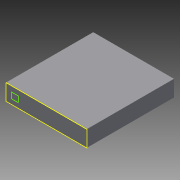
# Autodesk Inventor part: Five Pin Plug
Saved by Autodesk Inventor 2014 (Build 180170000, 170)
## iProperties
Created: 2014-02-26
Part Number: Five Pin Plug
Material: Generic
Document SubType Name: Modeling
Designer: Spooner
Density: 1 g/cm^3
Appearance: Default
Author: Spooner
Autodesk Inventor part; units mm, degrees
ref_plane "YZ Plane" through (0, 0, 0) normal (1, 0, 0) x (0, 1, 0)
ref_plane "XZ Plane" through (0, 0, 0) normal (0, 1, 0) x (-1, 0, 0)
ref_plane "XY Plane" through (0, 0, 0) normal (0, 0, 1) x (1, 0, 0)
sketch "Sketch1" plane through (0, 0, 0) normal (0, 1, 0) x (-1, 0, 0)
  line L0 (0, 0) -> (12.7, 0)
  line L1 (12.7, 0) -> (12.7, 13.716)
  line L2 (12.7, 13.716) -> (0, 13.716)
  line L3 (0, 13.716) -> (0, 0)
  dimension "d0" = 12.7
  dimension "d1" = 13.716
  constraints: 8 end point, 2 parallel, 1 horizontal, 1 perpendicular
  measures "d0" distance of L0.start L0.end
  measures "d1" distance of L2.end L0.start
extrude "Extrusion1" add sketch "Sketch1" along normal blind 2.54
sketch "Sketch2" plane through (-12.7, 0, 13.716) normal (0, 0, 1) x (1, 0, 0)
  line L0 (0, 0) -> (12.7, 0) projected
  line L1 (12.7, 0) -> (12.7, 2.54) projected
  line L2 (0, 2.54) -> (12.7, 2.54) projected
  line L3 (0, 0) -> (0, 2.54) projected
  line L4 (0.848, 1.7003) -> (1.893, 1.7003)
  line L5 (1.893, 1.7003) -> (1.893, 0.7782)
  line L6 (1.893, 0.7782) -> (0.848, 0.7782)
  line L7 (0.848, 0.7782) -> (0.848, 1.7003)
  constraints: 8 end point, 2 parallel, 1 horizontal, 1 perpendicular
body "Solid1"
